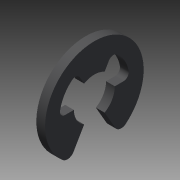
# Autodesk Inventor part: D-9770-rr
Saved by Autodesk Inventor 2014 (Build 180170000, 170)
## iProperties
Created: 2014-01-19
Part Number: D-9770-rr
Material: Generic
Catalog Web Link: www.cadenas.de
Description: Pivot Bracket for Original Line Cylinders - Retaining Ring-
Vendor: BIMBA
Document SubType Name: Standard Catalog Part
Designer: Michael
Manufacturer: BIMBA
Density: 1 g/cm^3
Appearance: RGB(84.00000259280115,84.00000259280115,84.00000259280115)
Category: PARTsolutions
Company: BIMBA
Title: D-9770-rr
Author: Cadenas PARTsolutions
PSOL_IDENT_0: {$CADENAS_DATA\23d-libs\bimba\bimba\bimba_imperial\bimba_full_line\original_line_cylinders\accessori
PSOL_IDENT_1: es\retaining_ring.prj},212 {VTYP=3D},{NB=D-9770-rr},{LINA=D-9770-rr},{NN=Pivot Bracket for Original
PSOL_IDENT_2: Line Cylinders - Retaining Ring},{DATE=06.12.2011 06:40:21},{GEOMDATE=06.12.2011 00:00:00},{VERSION=
PSOL_IDENT_3: },{LINEID=30},{LINESUBID=-1},{WBVAR=}  {NB=D-9770-rr},{LINA=D-9770-rr},{KT=DUMMY},{PN=D-9770},{MAT=Z
PSOL_IDENT_4: inc-Plated Carbon Steel},{D1=0.28200000},{W=0.11700000},{L=0.02500000},{D2=0.1995},{AN1=60.00000000}
PSOL_IDENT_5: ,{AN2=60.00000000},{R1=0.01500000},{R2=0.02000000},{BE=0}
CNS_NN: Pivot Bracket for Original Line Cylinders - Retaining Ring
CNS_NB: D-9770-rr
CNS_NBSYN: $PN.-rr
CNS_LINA: D-9770-rr
CNS_PN: D-9770
CNS_MAT: Zinc-Plated Carbon Steel
CNS_D1: 0.28200000
CNS_W: 0.11700000
CNS_L: 0.02500000
CNS_D2: 0.200
CNS_AN1: 60.00000000
CNS_AN2: 60.00000000
CNS_R1: 0.01500000
CNS_R2: 0.02000000
CNS_BE: 0
SUPPLIER: BIMBA
ARTICLENO: D-9770-rr
BOMINFO: D-9770-rr
CREATOR: CADENAS GmbH
Autodesk Inventor part; units mm, degrees
ref_plane "YZ Plane" through (0, 0, 0) normal (1, 0, 0) x (0, 1, 0)
ref_plane "XZ Plane" through (0, 0, 0) normal (0, 1, 0) x (-1, 0, 0)
ref_plane "XY Plane" through (0, 0, 0) normal (0, 0, 1) x (1, 0, 0)
sketch "Sketch_1" plane through (0, 0, 0) normal (1, 0, 0) x (0, 1, 0)
  arc A0 (-2.7629, -2.2787) -> (-2.7629, 2.2787) centre (0, 0) ccw
  arc A1 (-2.7629, 2.2787) -> (-2.625, 1.5156) centre (-2.371, 1.9555) ccw
  line L0 (-2.625, 1.5156) -> (-1.2868, 0.7429)
  arc A2 (0, 1.4859) -> (-1.2868, 0.7429) centre (0, 0) ccw
  line L1 (0, 1.4859) -> (0, 2.1187)
  arc A3 (0.4484, 2.4936) -> (0, 2.1187) centre (0.381, 2.1187) ccw
  arc A4 (1.9353, 1.6352) -> (0.4484, 2.4936) centre (0, 0) ccw
  arc A5 (1.8348, 1.0593) -> (1.9353, 1.6352) centre (1.6443, 1.3893) ccw
  line L2 (1.8348, 1.0593) -> (1.2868, 0.7429)
  arc A6 (1.2868, -0.7429) -> (1.2868, 0.7429) centre (0, 0) ccw
  line L3 (1.2868, -0.7429) -> (1.8348, -1.0593)
  arc A7 (1.9353, -1.6352) -> (1.8348, -1.0593) centre (1.6443, -1.3893) ccw
  arc A8 (0.4484, -2.4936) -> (1.9353, -1.6352) centre (0, 0) ccw
  arc A9 (0, -2.1187) -> (0.4484, -2.4936) centre (0.381, -2.1187) ccw
  line L4 (0, -2.1187) -> (0, -1.4859)
  arc A10 (-1.2868, -0.7429) -> (0, -1.4859) centre (0, 0) ccw
  line L5 (-1.2868, -0.7429) -> (-2.625, -1.5156)
  arc A11 (-2.625, -1.5156) -> (-2.7629, -2.2787) centre (-2.371, -1.9555) ccw
  constraints: 24 point on circle, 12 centre point, 12 end point
extrude "Extrusion1" add sketch "Sketch_1" along normal mid plane 0.635
ref_plane "rr_XY" through (0, 0, 0) normal (1, 0, 0) x (0, 0, -1)
ref_plane "rr_YZ" through (0, 0, 0) normal (0, 0, -1) x (0, 1, 0)
ref_plane "rr_ZX" through (0, 0, 0) normal (0, 1, 0) x (1, 0, 0)
body "Solid1"
